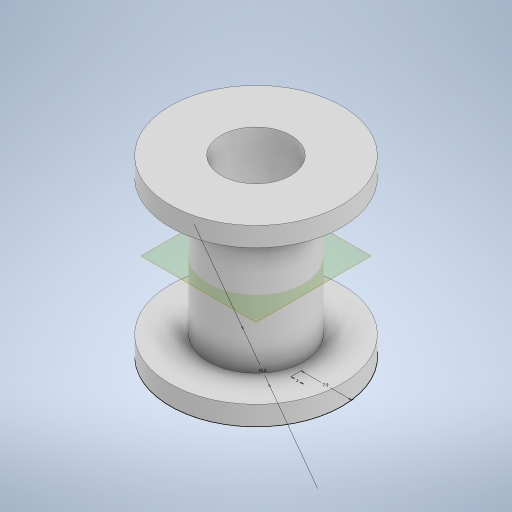
# Autodesk Inventor part: 코일감는부분(미니)
Saved by Autodesk Inventor 2023 (Build 270158000, 158)
## iProperties
Created: 2023-04-26
Part Number: 코일감는부분(미니)
Material: 일반
Document SubType Name: Modeling
Designer: rlatk
Density: 1 g/cm^3
Appearance: 기본값
Author: rlatk
Autodesk Inventor part; units mm, degrees
ref_plane "YZ Plane" through (0, 0, 0) normal (1, 0, 0) x (0, 1, 0)
ref_plane "XZ Plane" through (0, 0, 0) normal (0, 1, 0) x (-1, 0, 0)
ref_plane "XY Plane" through (0, 0, 0) normal (0, 0, 1) x (1, 0, 0)
sketch "스케치1" plane through (0, 0, 0) normal (0, 1, 0) x (-1, 0, 0)
  circle A0 centre (0, 0) radius 5.4
  circle A1 centre (0, 0) radius 13.3
  circle A2 centre (0, 0) radius 7.4
  dimension "d0" = 10.8
  dimension "d1" = 7.9
  dimension "d7" = 2
  constraints: 3 centre point, 1 coincident
  measures "d0" diameter of A0
  measures "d1" radial gap between concentric circles of A0 A1
  measures "d7" radial gap between concentric circles of A0 A2
extrude "돌출1" add sketch "스케치1" along normal blind 27 contours A0
extrude "돌출2" add sketch "스케치1" along normal blind 3 contours A1 | A2
ref_plane "작업 평면1" through (0, 13.5, 0) normal (0, -1, 0) x (1, 0, 0)
mirror "미러1" about plane through (0, 13.5, 0) normal (0, -1, 0) of "돌출2"
extrude "돌출3" add sketch "스케치1" along normal blind 27 contours A0 | A2
extrude "돌출4" cut sketch "스케치1" along normal blind 42 contours A0
